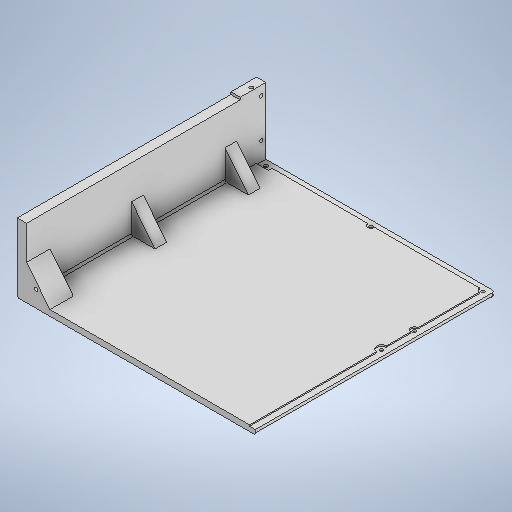
# Autodesk Inventor part: オンゲキボタン_bottom_right
Saved by Autodesk Inventor 2025.2 (Build 292293000, 293)
## iProperties
Created: 2025-05-16
Part Number: オンゲキボタン_bottom_right
Material: 一般
Document SubType Name: Modeling
Designer: mahhy
Density: 1 g/cm^3
Appearance: 既定
Author: mahhy
## iProperties of the stored document オンゲキボタン_bottom_right_3D プリント.ipt
Created: 2025-05-16
Part Number: オンゲキボタン_bottom_right_3D プリント
Material: 一般
Document SubType Name: Modeling
Designer: mahhy
Density: 1 g/cm^3
Appearance: 既定
Author: mahhy
Autodesk Inventor part; units mm, degrees
ref_plane "YZ Plane" through (0, 0, 0) normal (1, 0, 0) x (0, 1, 0)
ref_plane "XZ Plane" through (0, 0, 0) normal (0, 1, 0) x (-1, 0, 0)
ref_plane "XY Plane" through (0, 0, 0) normal (0, 0, 1) x (1, 0, 0)
sketch "スケッチ1" plane through (0, 0, 0) normal (0, 1, 0) x (-1, 0, 0)
  line L0 (0, 0) -> (204, 0)
  line L1 (204, 0) -> (204, -205)
  line L2 (204, -205) -> (0, -205)
  line L3 (0, -205) -> (0, 0)
  dimension "d0" = 204
  dimension "d1" = 205
  constraints: 8 end point, 2 parallel, 1 horizontal, 1 perpendicular
  measures "d0" distance of L1.end L2.end
  measures "d1" distance of L0.end L1.end
extrude "押し出し1" add sketch "スケッチ1" along normal blind 5
sketch "スケッチ2" plane through (0, 5, 0) normal (0, 1, 0) x (1, 0, 0)
  line L0 (-204, 205) -> (-204, 0) projected
  line L1 (0, 205) -> (-204, 205) projected
  line L2 (-204, 0) -> (-196, 0)
  line L3 (-196, 0) -> (-196, 205)
  line L4 (-196, 205) -> (-204, 205)
  line L5 (-204, 205) -> (-204, 0)
  point P0 (0, 0)
  dimension "d4" = 8
  constraints: 8 end point, 2 parallel, 1 horizontal, 1 perpendicular, 1 point on line
  measures "d4" distance of L4.end L3.end
extrude "押し出し2" add sketch "スケッチ2" along normal blind 56
sketch "スケッチ3" plane through (0, 61, 0) normal (0, 1, 0) x (1, 0, 0)
  line L0 (-204, 205) -> (-204, 0) projected
  line L1 (-196, 0) -> (-196, 205) projected
  line L2 (-204, 0) -> (-196, 0)
  line L3 (-196, 0) -> (-196, 183)
  line L4 (-196, 183) -> (-204, 183)
  line L5 (-204, 183) -> (-204, 0)
  line L6 (-196, 205) -> (-204, 205) projected
  point P0 (0, 0)
  point P1 (-200, 183)
  dimension "d7" = 22
  constraints: 8 end point, 2 parallel, 1 horizontal, 1 midpoint, 1 perpendicular, 1 point on line
  measures "d7" distance from line of L6 point (-200, 183)
extrude "押し出し3" cut sketch "スケッチ3" against normal blind 2 contours L4 L1 L2 L0
sketch "スケッチ4" plane through (0, 61, 0) normal (0, 1, 0) x (1, 0, 0)
  circle A0 centre (-198.5, 195) radius 1.5
  line L0 (-196, 205) -> (-204, 205) projected
  line L1 (-196, 183) -> (-196, 205) projected
  line L2 (-204, 205) -> (-204, 183) projected
  point P0 (0, 0)
  dimension "d10" = 3
  dimension "d11" = 10
  dimension "d13" = 5.5
  constraints: 1 centre point
  measures "d10" diameter of A0
  measures "d11" distance from line of L0 A0.centre
  measures "d13" distance from line of L2 A0.centre
extrude "押し出し4" cut sketch "スケッチ4" against normal blind 10
sketch "スケッチ5" plane through (-204, 0, -205) normal (-1, 0, 0) x (0, 0, 1)
  circle A0 centre (4, 53) radius 1.5
  circle A1 centre (4, 20) radius 1.5
  line L0 (0, 61) -> (22, 61) projected
  line L1 (0, 0) -> (0, 61) projected
  point P0 (205, 0)
  dimension "d16" = 3
  dimension "d17" = 3
  dimension "d18" = 8
  dimension "d19" = 33
  dimension "d24" = 4
  constraints: 2 centre point, 1 vertical alignment
  measures "d16" diameter of A0
  measures "d17" diameter of A1
  measures "d18" distance from line of L0 A0.centre
  measures "d19" distance of A0.centre A1.centre
  measures "d24" distance from line of L1 A0.centre
extrude "押し出し5" cut sketch "スケッチ5" against normal blind 10
sketch "スケッチ6" plane through (-204, 0, -205) normal (-1, 0, 0) x (0, 0, 1)
  circle A0 centre (4, 53) radius 1.5 projected
  circle A1 centre (4, 53) radius 2.8
  circle A2 centre (4, 20) radius 1.5 projected
  circle A3 centre (4, 20) radius 2.8
  point P0 (205, 0)
  dimension "d22" = 5.6
  dimension "d23" = 5.6
  constraints: 2 centre point, 2 coincident
  measures "d22" diameter of A1
  measures "d23" diameter of A3
extrude "押し出し6" cut sketch "スケッチ6" against normal blind 2.5
sketch "スケッチ7" plane through (0, 0, 0) normal (0, -1, 0) x (1, 0, 0)
  circle A0 centre (-191, -200) radius 1.5
  circle A1 centre (-101, -200) radius 1.5
  circle A2 centre (-5, -200) radius 1.5
  line L0 (-204, 0) -> (0, 0) projected
  line L1 (0, 0) -> (0, -205) projected
  circle A3 centre (-5, -141) radius 1.5
  circle A4 centre (-5, -113) radius 1.5
  line L2 (0, -205) -> (-204, -205) projected
  dimension "d27" = 3
  dimension "d28" = 3
  dimension "d29" = 3
  dimension "d31" = 5
  dimension "d32" = 96
  dimension "d33" = 90
  dimension "d34" = 3
  dimension "d36" = 3
  dimension "d37" = 5
  dimension "d38" = 59
  dimension "d39" = 28
  constraints: 5 centre point, 2 horizontal alignment, 2 vertical alignment
  measures "d27" diameter of A0
  measures "d28" diameter of A1
  measures "d29" diameter of A2
  measures "d31" distance from line of L1 A2.centre
  measures "d32" distance of A2.centre A1.centre
  measures "d33" distance of A1.centre A0.centre
  measures "d34" diameter of A3
  measures "d36" diameter of A4
  measures "d37" distance from line of L2 A2.centre
  measures "d38" distance of A2.centre A3.centre
  measures "d39" distance of A4.centre A3.centre
extrude "押し出し7" cut sketch "スケッチ7" against normal through all
sketch "スケッチ8" plane through (0, 0, 0) normal (0, -1, 0) x (1, 0, 0)
  circle A0 centre (-5, -113) radius 1.5 projected
  circle A1 centre (-5, -113) radius 2.8
  circle A2 centre (-5, -141) radius 1.5 projected
  circle A3 centre (-5, -141) radius 2.8
  circle A4 centre (-5, -200) radius 1.5 projected
  circle A5 centre (-5, -200) radius 2.8
  circle A6 centre (-101, -200) radius 1.5 projected
  circle A7 centre (-101, -200) radius 2.8
  circle A8 centre (-191, -200) radius 1.5 projected
  circle A9 centre (-191, -200) radius 2.8
  point P0 (0, 0)
  dimension "d42" = 5.6
  dimension "d43" = 5.6
  dimension "d44" = 5.6
  dimension "d45" = 5.6
  dimension "d46" = 5.6
  constraints: 5 centre point, 5 coincident
  measures "d42" diameter of A1
  measures "d43" diameter of A3
  measures "d44" diameter of A5
  measures "d45" diameter of A7
  measures "d46" diameter of A9
extrude "押し出し8" cut sketch "スケッチ8" against normal blind 2.5
sketch "スケッチ9" plane through (0, 5, 0) normal (0, 1, 0) x (1, 0, 0)
  line L0 (0, 205) -> (-204, 205) projected
  line L1 (0, 0) -> (-5, 0)
  line L2 (-5, 0) -> (-5, 205)
  line L3 (-5, 205) -> (0, 205)
  line L4 (0, 205) -> (0, 0)
  line L5 (-196, 183) -> (-196, 205) projected
  line L6 (0, 205) -> (-196, 205)
  line L7 (-196, 205) -> (-196, 200)
  line L8 (-196, 200) -> (0, 200)
  line L9 (0, 200) -> (0, 205)
  circle A0 centre (-5, 141) radius 1.5 projected
  circle A1 centre (-5, 141) radius 3.1
  circle A2 centre (-5, 113) radius 1.5 projected
  circle A3 centre (-5, 113) radius 4.1
  circle A4 centre (-5, 200) radius 1.5 projected
  circle A5 centre (-5, 200) radius 3.1
  line L10 (-196, 205) -> (-185.8, 205)
  line L11 (-185.8, 205) -> (-185.8, 196.8)
  line L12 (-185.8, 196.8) -> (-196, 196.8)
  line L13 (-196, 196.8) -> (-196, 205)
  circle A6 centre (-101, 200) radius 1.5 projected
  circle A7 centre (-101, 200) radius 3.1
  point P0 (-5, 137.9)
  point P1 (-5, 117.1)
  point P2 (-5, 108.9)
  point P3 (-185.8, 200)
  point P4 (-8.1, 200)
  point P5 (-5, 196.9)
  point P6 (-5, 144.1)
  point P7 (-104.1, 200)
  point P8 (-97.9, 200)
  point P9 (-99.5, 200)
  point P10 (-102.5, 200)
  dimension "d49" = 5
  dimension "d50" = 5
  dimension "d51" = 6.2
  dimension "d52" = 8.2
  dimension "d53" = 6.2
  dimension "d54" = 10.2
  dimension "d55" = 8.2
  dimension "d58" = 6.2
  constraints: 24 end point, 6 parallel, 4 centre point, 4 coincident, 3 horizontal, 3 perpendicular, 2 point on line
  measures "d49" distance of L2.end L3.end
  measures "d50" distance of L7.end L6.end
  measures "d51" diameter of A1
  measures "d52" diameter of A3
  measures "d53" diameter of A5
  measures "d54" distance of L11.end L12.end
  measures "d55" distance of L10.end L11.end
  measures "d58" diameter of A7
extrude "押し出し9" cut sketch "スケッチ9" against normal blind 1 contours L4 L8 A5 L2 L0 | L2 A5 L8 A7 L11 L0 | L4 L1 L2 A3 A1 A5 L8 | L11 L8 L5 L0 | A5 L8 A4 L2 | L2 A4 L8 A5 | A5 L2 A4 L8 | L11 L12 L5 L8 | A4 L8 L2 | L2 L8 A4 | L8 A4 L2 A5 | A4 L2 L8 | A7 L8 A6 | L8 A6 A7 | L2 A4 L8 | A3 L2 A2 | L2 A2 A3 | A1 L2 A0 | L2 A0 A1 | A6 L8 | A2 L2 | L2 A2 | A0 L2 | L2 A0 picked at (-100.9397, 200.4964)
sketch "スケッチ10" plane through (0, 5, 0) normal (0, 1, 0) x (1, 0, 0)
  line L0 (-196, 0) -> (-176, 0)
  line L1 (-176, 0) -> (-176, 20)
  line L2 (-176, 20) -> (-196, 20)
  line L3 (-196, 20) -> (-196, 0)
  line L4 (-196, 196.8) -> (-196, 0) projected
  line L5 (-196, 90) -> (-176, 90)
  line L6 (-176, 90) -> (-176, 100)
  line L7 (-176, 100) -> (-196, 100)
  line L8 (-196, 100) -> (-196, 90)
  line L9 (-196, 170) -> (-176, 170)
  line L10 (-176, 170) -> (-176, 180)
  line L11 (-176, 180) -> (-196, 180)
  line L12 (-196, 180) -> (-196, 170)
  point P0 (0, 0)
  dimension "d59" = 20
  dimension "d60" = 20
  dimension "d61" = 20
  dimension "d62" = 10
  dimension "d63" = 70
  dimension "d64" = 20
  dimension "d65" = 10
  dimension "d66" = 70
  constraints: 24 end point, 6 parallel, 3 horizontal, 3 perpendicular, 2 point on line, 1 coincident
  measures "d59" distance of L2.end L1.end
  measures "d60" distance of L1.end L0.end
  measures "d61" distance of L7.end L6.end
  measures "d62" distance of L6.end L5.end
  measures "d63" distance between parallel lines of L2 L5
  measures "d64" distance of L11.end L10.end
  measures "d65" distance of L10.end L9.end
  measures "d66" distance between parallel lines of L9 L7
extrude "押し出し10" add sketch "スケッチ10" along normal blind 25
sketch "スケッチ11" plane through (-204, 0, 0) normal (0, 0, 1) x (1, 0, 0)
  line L0 (8, 30) -> (8, 5) projected
  line L1 (28, 5) -> (28, 30) projected
  line L2 (8, 30) -> (28, 5)
  line L3 (28, 5) -> (28, 30)
  line L4 (28, 30) -> (8, 30)
  point P0 (204, 0)
  constraints: 6 end point, 1 collinear, 1 perpendicular
extrude "押し出し11" cut sketch "スケッチ11" against normal through all
sketch "スケッチ12" plane through (-204, 0, 0) normal (0, 0, 1) x (1, 0, 0)
  circle A0 centre (16, 14) radius 1.5
  line L0 (0, 0) -> (0, 59) projected
  line L1 (8, 30) -> (8, 5) projected
  line L2 (8, 5) -> (28, 5) projected
  point P0 (204, 0)
  dimension "d71" = 3
  dimension "d73" = 8
  dimension "d74" = 9
  constraints: 1 centre point
  measures "d71" diameter of A0
  measures "d73" distance from line of L1 A0.centre
  measures "d74" distance from line of L2 A0.centre
extrude "押し出し12" cut sketch "スケッチ12" against normal blind 25
fillet "フィレット1" radius 2 2 edges at (-204, 30.5, -205) (0, 2, -205)
fillet "フィレット2" radius 1.5 4 edges at (-203.4142, 0, -204.4142) (-102, 0, -205) (-204, 0, -101.5) (0, 0, -101.5)
fillet "フィレット3" radius 1.5 2 edges at (-196, 5, -135) (-196, 5, -55)
